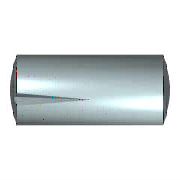
# Autodesk Inventor part: ISO 8745 - 2 x 10
Saved by Autodesk Inventor 2023.1 (Build 271208000, 208)
## iProperties
IsCustomPart: 0
Created: 2021-02-02
Part Number: ISO 8745 - 2 x 10
Material: Edelstahl, austenitisch
Description: Kerbstift
Document SubType Name: Modeling
Standard: ISO 8745
Designer: rYan
Standards Organization: DIN
Language: de-DE
Size Designation: 2 x 10
Categories: <MemberInstance><Categories><Category DisplayName="Verbindungselemente" InternalName="e4da775c-781d-43d5-af7c-5136215cf5a6" Mnemonic="FSTN"><Category DisplayName="Stifte" InternalName="3b3d1810-ac9b-4ede-8c7f-cc6b956350b0" Mnemonic="PIN"><CategoryParameter DisplayName="Nenndurchmesser" InternalName="6cc331d7-8ea1-4fca-9c9a-55ec966217e5" Mnemonic="nomdia"/><CategoryParameter DisplayName="Nennlänge" InternalName="897bd938-6adf-4e3c-a2d4-0d7cae45eecd" Mnemonic="nomlen"/><Category DisplayName="Gekerbt" InternalName="f15d0e3b-3a02-454e-afff-cb37befcf7c5" Mnemonic="NLPIN"><CategoryParameter DisplayName="Typ" InternalName="67addd20-41fb-4872-ba94-3c8eeb37a4c0" Mnemonic="type"/><CategoryParameter DisplayName="Funktionslänge" InternalName="d4136c1f-288c-40f8-9651-e7f7ed6303af" Mnemonic="fnclen"/><Category DisplayName="Zylinderkerbstifte ohne Kopf" InternalName="87d2efa0-d970-4bf0-8358-3eec02ada24b" Mnemonic="NLPINBH"/></Category></Category></Category><Category DisplayName="Datentyp" InternalName="23b78d0f-2648-40c6-8793-ca6db495c9e8" Mnemonic="DATATYPE"><CategoryParameter DisplayName="Anzeigename" InternalName="05415f3d-3907-474b-a020-eb9d644f4cf3" Mnemonic="DISPLAYNAME"/><CategoryParameter DisplayName="Norm" InternalName="0c0a119c-1e12-4c84-803f-101930972f5e" Mnemonic="STANDARD"/><CategoryParameter DisplayName="Beschreibung" InternalName="13903e3d-64b1-4950-80da-f627842ea37f" Mnemonic="DESCRIPTION"/><CategoryParameter DisplayName="Bezeichnung" InternalName="2675968c-4ce5-49e0-a4f5-552d29089031" Mnemonic="DESIGNATION"/><CategoryParameter DisplayName="Standardzeile" InternalName="2af9ec52-faaa-4026-b378-f9fa4afca842" Mnemonic="DEFAULTROW"/><CategoryParameter DisplayName="Ordnername" InternalName="3f06958e-8713-4116-9be7-ed6184ecc97b" Mnemonic="FOLDERNAME"/><CategoryParameter DisplayName="Revisionsanleitung" InternalName="45a75005-10b1-4dfc-8d6d-dfe629f0b93c" Mnemonic="REVISIONGUID"/><CategoryParameter DisplayName="Dateiname" InternalName="8b46a4cc-9585-4fed-90c3-899f57e09a73" Mnemonic="FILENAME"/><CategoryParameter DisplayName="Normungsorganisation" InternalName="8f5914e1-4693-403f-8ab5-d37768198c9d" Mnemonic="STDSORG"/><CategoryParameter DisplayName="Gruppenversion" InternalName="914462f6-6e19-4b14-ba84-155b9680b1d0" Mnemonic="FAMILYREVISION"/><CategoryParameter DisplayName="Normrevision" InternalName="91d5a463-65c2-4fde-b823-3b7fea5e8e17" Mnemonic="STANDARDREVISION"/><CategoryParameter DisplayName="Variantenrevision" InternalName="a65d44b9-392f-4f4f-857b-e4b3d54996fe" Mnemonic="MEMBERREVISION"/><CategoryParameter DisplayName="ClipFormat" InternalName="bc51e27b-3422-4e78-93ef-cec197ddf230" Mnemonic="CLIPFORMAT"/><CategoryParameter DisplayName="Hersteller" InternalName="cd6c7a72-a28a-4e50-99a9-2c7f4e13e5ad" Mnemonic="MANUFACTURER"/><CategoryParameter DisplayName="InternerName" InternalName="cf1d0246-76d9-4b4a-8305-fa0409afb5c1" Mnemonic="INTERNALNAME"/><CategoryParameter DisplayName="IstMetrisch" InternalName="e2385c5b-1ea4-4823-96a8-8de651266ec3" Mnemonic="ISMETRIC"/><Category DisplayName="Bauteil" InternalName="c0e0b642-3bcb-4cc8-9e80-f96d35c4afa4" Mnemonic="PART"><CategoryParameter DisplayName="Bauteilnummer" InternalName="016b6077-bfbe-49bd-92c9-d8d59c39c941" Mnemonic="PARTNUMBER"/><CategoryParameter DisplayName="Bestandsnummer" InternalName="4dba7c1c-e26c-444e-836c-b08b433409a8" Mnemonic="STOCKNUMBER"/><CategoryParameter DisplayName="Materialschlüssel" InternalName="5c9a8adb-dd2b-4535-b97f-0a94a95fe41f" Mnemonic="MATERIALKEY"/><CategoryParameter DisplayName="Material" InternalName="818a152a-d3c3-49ca-80ee-df7d91421b8e" Mnemonic="MATERIAL"/></Category></Category><Category DisplayName="Abwärtskompatibilitätszuordnung DA" InternalName="924fff40-ddd0-4eff-ad42-30e3774ef79e" Mnemonic="LEGACYMAPDA"><CategoryParameter DisplayName="DA-Cookie" InternalName="316934ee-8fe1-4c7a-9c36-f2d79e1add1a" Mnemonic="DACOOKIE"/></Category><Category DisplayName="ÄltereVersionenzuweisen" InternalName="cd87c42b-3e48-431e-b5c0-1cbeb14dfe77" Mnemonic="LEGACYMAP"><CategoryParameter DisplayName="Eindeutige DA-Varianten-ID" InternalName="0918ad47-427f-4fed-ae26-24c81c58f590" Mnemonic="DACOOKIE"/><CategoryParameter DisplayName="ID zusammenführen" InternalName="0ee8fb18-e2ed-4f39-96f6-1f4b5f50aa71" Mnemonic="MERGE11"/><CategoryParameter DisplayName="Eindeutige CC-Varianten-ID" InternalName="5193edd4-b2b0-4ab4-9d54-de900eee34e0" Mnemonic="CCCOOKIE"/><CategoryParameter DisplayName="ID aufteilen" InternalName="72b5c83c-be7f-45c4-ae51-9160ea6deb26" Mnemonic="SPLIT"/><CategoryParameter DisplayName="VarianteID" InternalName="8e5e0294-fc51-4c8f-b3d7-003dc5ed94f6" Mnemonic="MEMBERID"/><CategoryParameter DisplayName="Katalogname" InternalName="d99d1e27-aa94-4de2-af4c-c348882a6f4f" Mnemonic="CATALOGNAME"/><CategoryParameter DisplayName="Gruppennummer" InternalName="e705e1f4-09cb-413e-91f9-551b4188271e" Mnemonic="FAMILYNUMBER"/></Category></Categories><FamilyTemplate Id="si0083"><FamilyTemplateParameters><FamilyTemplateParameter ObjectType="kUserParameterObject" ValueType="xs:double" Id="1" ObjectReferenceKey="NND1"/><FamilyTemplateParameter ObjectType="kUserParameterObject" ValueType="xs:double" Id="2" ObjectReferenceKey="NND"/><FamilyTemplateParameter ObjectType="kUserParameterObject" ValueType="xs:double" Id="3" ObjectReferenceKey="KAH"/><FamilyTemplateParameter ObjectType="kUserParameterObject" ValueType="xs:double" Id="4" ObjectReferenceKey="NLG"/><FamilyTemplateParameter ObjectType="kUserParameterObject" ValueType="xs:double" Id="5" ObjectReferenceKey="FAC"/><FamilyTemplateParameter ObjectType="kUserParameterObject" ValueType="xs:double" Id="6" ObjectReferenceKey="NLG1"/><FamilyTemplateParameter ObjectType="kPropertyObject" ValueType="xs:string" Id="100" ObjectReferenceKey="{32853F0F-3444-11d1-9E93-0060B03C1CA6}" SubObjectId="52"/><FamilyTemplateParameter ObjectType="kPropertyObject" ValueType="xs:string" Id="105" ObjectReferenceKey="{32853F0F-3444-11d1-9E93-0060B03C1CA6}" SubObjectId="5"/><FamilyTemplateParameter ObjectType="kPartComponentDefinitionObject" ValueType="xs:string" Id="110" SubObjectId="Material"/></FamilyTemplateParameters></FamilyTemplate><CategoryParameterMap><ParamToTemplateMap><ParamToTemplate CategoryParameter="//CategoryParameter[@InternalName='05415f3d-3907-474b-a020-eb9d644f4cf3']" ConstantValue="DIN EN ISO 8745"/><ParamToTemplate CategoryParameter="//CategoryParameter[@InternalName='cf1d0246-76d9-4b4a-8305-fa0409afb5c1']" ConstantValue="f76ecf70-8102-4cec-95be-df48fe5ae94a"/><ParamToTemplate CategoryParameter="//CategoryParameter[@InternalName='3f06958e-8713-4116-9be7-ed6184ecc97b']" ConstantValue="ISO 8745(2)"/><ParamToTemplate CategoryParameter="//CategoryParameter[@InternalName='914462f6-6e19-4b14-ba84-155b9680b1d0']" ConstantValue="10"/><ParamToTemplate CategoryParameter="//CategoryParameter[@InternalName='bc51e27b-3422-4e78-93ef-cec197ddf230']" ConstantValue="CF_INVENTOR.STDPARTS"/><ParamToTemplate CategoryParameter="//CategoryParameter[@InternalName='e2385c5b-1ea4-4823-96a8-8de651266ec3']" ConstantValue="true"/><ParamToTemplate CategoryParameter="//CategoryParameter[@InternalName='13903e3d-64b1-4950-80da-f627842ea37f']" ConstantValue="Grooved Pin"/><ParamToTemplate CategoryParameter="//CategoryParameter[@InternalName='8f5914e1-4693-403f-8ab5-d37768198c9d']" ConstantValue="DIN"/><ParamToTemplate CategoryParameter="//CategoryParameter[@InternalName='0c0a119c-1e12-4c84-803f-101930972f5e']" ConstantValue="ISO 8745"/><ParamToTemplate CategoryParameter="//CategoryParameter[@InternalName='cd6c7a72-a28a-4e50-99a9-2c7f4e13e5ad']" TemplateParameter="104"/><ParamToTemplate CategoryParameter="//CategoryParameter[@InternalName='91d5a463-65c2-4fde-b823-3b7fea5e8e17']" TemplateParameter="103"/><ParamToTemplate CategoryParameter="//CategoryParameter[@InternalName='45a75005-10b1-4dfc-8d6d-dfe629f0b93c']" ConstantValue="e5327a38-073d-4733-bf9d-12eeab7edc42"/><ParamToTemplate CategoryParameter="//CategoryParameter[@InternalName='2af9ec52-faaa-4026-b378-f9fa4afca842']" ConstantValue="10"/><ParamToTemplate CategoryParameter="//CategoryParameter[@InternalName='d99d1e27-aa94-4de2-af4c-c348882a6f4f']" ConstantValue="DIN"/><ParamToTemplate CategoryParameter="//CategoryParameter[@InternalName='e705e1f4-09cb-413e-91f9-551b4188271e']" ConstantValue="211"/><ParamToTemplate CategoryParameter="//CategoryParameter[@InternalName='8b46a4cc-9585-4fed-90c3-899f57e09a73']" ConstantValue="ISO 8745 - 2 x 10(6)"/><ParamToTemplate CategoryParameter="//CategoryParameter[@InternalName='a65d44b9-392f-4f4f-857b-e4b3d54996fe']" ConstantValue="44ED0D85-0CAA-4E11-BC16-1B02BBF9B82E"/><ParamToTemplate CategoryParameter="//CategoryParameter[@InternalName='d4136c1f-288c-40f8-9651-e7f7ed6303af']" ConstantValue="9,5"/><ParamToTemplate CategoryParameter="//CategoryParameter[@InternalName='8e5e0294-fc51-4c8f-b3d7-003dc5ed94f6']" ConstantValue="90"/><ParamToTemplate CategoryParameter="//CategoryParameter[@InternalName='316934ee-8fe1-4c7a-9c36-f2d79e1add1a']" ConstantValue="*Din~I8745~2x10-St~10~DIN 1472*"/><ParamToTemplate CategoryParameter="//CategoryParameter[@InternalName='2675968c-4ce5-49e0-a4f5-552d29089031']" TemplateParameter="100"/><ParamToTemplate CategoryParameter="//CategoryParameter[@InternalName='818a152a-d3c3-49ca-80ee-df7d91421b8e']" TemplateParameter="110"/><ParamToTemplate CategoryParameter="//CategoryParameter[@InternalName='897bd938-6adf-4e3c-a2d4-0d7cae45eecd']" TemplateParameter="4"/><ParamToTemplate CategoryParameter="//CategoryParameter[@InternalName='6cc331d7-8ea1-4fca-9c9a-55ec966217e5']" TemplateParameter="2"/><ParamToTemplate CategoryParameter="//CategoryParameter[@InternalName='016b6077-bfbe-49bd-92c9-d8d59c39c941']" TemplateParameter="105"/></ParamToTemplateMap></CategoryParameterMap></MemberInstance>
Density: 8 g/cm^3
Appearance: Halbpoliert
Author: rYan
Autodesk Inventor part; units mm, degrees
ref_plane "YZ Plane" through (0, 0, 0) normal (1, 0, 0) x (0, 1, 0)
sketch "Skizze1" plane through (0, 0, 0) normal (0, 0, 1) x (1, 0, 0)
  line L0 (0, 0) -> (10, 0)
  line L1 (0.25, 1) -> (9.75, 1)
  arc A0 (0.25, 1) -> (0, 0) centre (2.125, 0) ccw
  arc A1 (10, 0) -> (9.75, 1) centre (7.875, 0) ccw
  line L2 (10, 0) -> (10, 0.84) construction
  line L3 (10, 0.84) -> (5, 1) construction
  line L4 (-12.8617, 0) -> (72.8617, 0) projected
  line L5 (0, 12.1847) -> (0, -2.0308) projected
  point P0 (5, 0)
  dimension "d0" = 2
  dimension "d1" = 10
  dimension "d2" = 1.68
  dimension "d12" = 5
  dimension "d17" = 0.25
  dimension "d18" = 0.25
  constraints: 8 end point, 4 point on circle, 3 point on line, 2 centre point, 2 midpoint, 1 coincident, 1 horizontal, 1 parallel, 1 tangent
  measures "d0" diameter of L1 L0
  measures "d1" distance of L0.end L0.start
  measures "d2" diameter of L2.end L0
  measures "d12" horizontal distance of L2.end L3.end
  measures "d17" horizontal distance of L1.start point (0, 0)
  measures "d18" horizontal distance of L0.end L1.end
revolve "Körper" add sketch "Skizze1" angle 360 about axis through (0, 0, 0) along (1, 0, 0)
ref_plane "Work Plane1" through (10, 0, 0) normal (1, 0, 0) x (0, 1, 0)
sketch "Skizze2" plane through (10, 0, 0) normal (1, 0, 0) x (0, 1, 0)
  line L0 (0, -14) -> (0, 14) projected
ref_plane "Work Plane2" through (10, 0, -10) normal (0.9995, -0.032, 0) x (0.032, 0.9995, 0)
sketch "Skizze3" plane through (10, 0, -10) normal (0.9995, -0.032, 0) x (0.032, 0.9995, 0)
  ellipse E0 centre (-0.008, 10) end of major axis (-0.008, 11) minor radius 0.9995 projected
  line L0 (-0.1599, 10) -> (0.8396, 10) projected
  line L1 (0.8396, 10) -> (0.9862, 10.1027)
  line L2 (0.8396, 10) -> (0.9862, 9.8973)
  arc A0 (0.9862, 9.8973) -> (0.9862, 10.1027) centre (-0.008, 10) ccw
  dimension "d7" = 70
  constraints: 4 end point, 2 point on circle, 1 centre point, 1 coincident, 1 symmetric about line, 3 other
  measures "d7" angle of L1 L2
extrude "Nut" cut sketch "Skizze3" against normal up to next contours L2 L1 E0 picked at (0.9387, 9.9486)
pattern_circular "Nuten" count 3 over 360 about axis through (5, 0, 0) along (1, 0, 0) of "Nut"
equation "\"d0\" = NND"
equation "\"d1\" = NLG"
equation "\"d2\" = 0.84 * NND"
equation "\"d17\" = KAH"
equation "\"d18\" = KAH"
equation "\"d8\" = 0.5 * NLG"
equation "\"NND\" = 2"
equation "\"NLG\" = 10"
equation "\"KAH\" = 0.25"
equation "\"d6\" = -d5"
equation "\"FAC\" = 0.5"
equation "\"NND1\" = 2.15"
equation "\"NLG1\" = 9.5"
body "Solid1"
